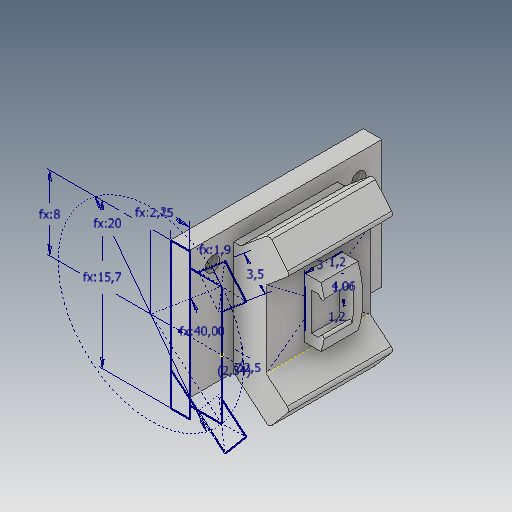
# Autodesk Inventor part: IMU_Fixation
Saved by Autodesk Inventor 2021.4 (Build 254397000, 397)
## iProperties
Created: 2022-04-26
Part Number: IMU_Fixation
Material: Generisch
Document SubType Name: Modeling
Designer: alexw
Density: 1 g/cm^3
Appearance: Vorgabe
Mass: 1.28857 g
Surface Area: 10.9165 cm^2
Volume: 1.28857 cm^3
SledWidth: 3,500 mm
SledDepth: 1,900 mm
Author: alexw
Autodesk Inventor part; units mm, degrees
ref_plane "YZ Plane" through (0, 0, 0) normal (1, 0, 0) x (0, 1, 0)
sketch "Sketch1" plane through (0, 0, 0) normal (0, 0, 1) x (1, 0, 0)
  line L0 (-1, 8) -> (1, 8)
  line L1 (1, 8) -> (1, -7.7)
  line L2 (1, -7.7) -> (-1, -7.7)
  line L3 (-1, -7.7) -> (-1, 8)
  line L4 (-1, 0) -> (1, 0) construction
  circle A0 centre (-3.15, 0) radius 10 construction
  line L5 (1, -6.4279) -> (4.5104, -6.4279)
  line L6 (4.5104, -6.4279) -> (4.5104, 6.4279)
  line L7 (4.5104, 6.4279) -> (1, 6.4279)
  line L8 (1, 6.4279) -> (1, -6.4279)
  line L9 (-3.15, 0) -> (4.5104, 6.4279) construction
  line L10 (-3.15, 0) -> (4.5104, -6.4279) construction
  line L11 (4.1798, 3.866) -> (7.0908, 6.3086) construction
  line L12 (7.0908, 6.3086) -> (4.8411, 8.9898)
  line L13 (4.8411, 8.9898) -> (1.9301, 6.5472) construction
  line L14 (1.9301, 6.5472) -> (4.1798, 3.866) construction
  line L15 (4.1798, 3.866) -> (4.8411, 8.9898) construction
  line L16 (7.0908, 6.3086) -> (1.9301, 6.5472) construction
  line L17 (4.1798, -3.866) -> (7.0908, -6.3086) construction
  line L18 (7.0908, -6.3086) -> (4.8411, -8.9898)
  line L19 (4.8411, -8.9898) -> (1.9301, -6.5472) construction
  line L20 (1.9301, -6.5472) -> (4.1798, -3.866) construction
  line L21 (4.1798, -3.866) -> (4.8411, -8.9898) construction
  line L22 (7.0908, -6.3086) -> (1.9301, -6.5472) construction
  line L23 (4.8411, 8.9898) -> (1.7879, 6.4279)
  line L24 (7.0908, 6.3086) -> (4.5104, 4.1434)
  line L25 (7.0908, -6.3086) -> (4.5104, -4.1434)
  line L26 (4.8411, -8.9898) -> (1.7879, -6.4279)
  line L27 (1, -6.4279) -> (1.7879, -6.4279)
  line L28 (1, -5.7667) -> (1, -6.4279)
  line L29 (1.7879, -6.4279) -> (-1, -4.0885)
  line L30 (6.85, 0) -> (-3.15, 0) construction
  point P0 (0, 0)
  point P1 (0, 0)
  point P2 (1.7879, 6.4279)
  point P3 (1, 6.4279)
  point P4 (1, -6.4279)
  point P5 (1.7879, -6.4279)
  point P6 (1, -5.7667)
  point P7 (6.7716, 1.25)
  dimension "d0" = 15.7
  dimension "d3" = 20
  dimension "SledAngle" = 40
  dimension "SledWidth" = 3.5
  dimension "SledDepth" = 1.9
  dimension "d7" = 2
  dimension "d30" = 2.15
  dimension "d74" = 8
  dimension "d88" = 2.3396
  dimension "d89" = 2.5
  constraints: 62 end point, 14 point on line, 7 parallel, 6 midpoint, 5 perpendicular, 4 horizontal, 4 symmetric about line, 3 point on circle, 1 centre point, 1 coincident
  measures "d0" distance of L2.end L0.start
  measures "d3" diameter of A0
  measures "SledAngle" angle of L4 L9
  measures "SledWidth" distance between parallel lines of L11 L13
  measures "SledDepth" distance from line of L12 L6.end
  measures "d7" distance of L0.start L0.end
  measures "d30" distance from line of L3 L9.start
  measures "d74" distance between parallel lines of L0 L4
  measures "d88" distance edge to line of A0 L6
  measures "d89" diameter of point (6.772, 1.25) L30
extrude "Extrusion1" add sketch "Sketch1" against normal blind 20.8 contours L0 L1 L29 L3
ref_plane "Work Plane1" through (0, 0, -4.8) normal (0, 0, 1) x (1, 0, 0)
ref_plane "Work Plane2" through (0, 0, -16) normal (0, 0, -1) x (-1, 0, 0)
extrude "Sled1" add sketch "Sketch1" against normal blind 3 from surface at -4.8 contours L7 L6 L5 L29 L1 | L23 L12 L24 L6 L7 | L5 L6 L25 L18 L26
extrude "Extrusion8" add sketch "Sketch1" along normal blind 3 from surface at -16 contours L7 L6 L5 L29 L1 | L23 L12 L24 L6 L7 | L5 L6 L25 L18 L26
sketch "Sketch4" plane through (-1, -4.0885, 0) normal (-1, 0, 0) x (0, 0, 1)
  line L0 (-24.96, 4.0885) -> (4.16, 4.0885) construction
  line L1 (-18.3, 9.5885) -> (-2.5, 9.5885) construction
  line L2 (0, 12.0885) -> (-20.8, 12.0885) construction
  line L3 (-10.4, 12.0885) -> (-10.4, 9.5885) construction
  point P0 (0, 4.0885)
  point P1 (-2.5, -1.4115)
  point P2 (-18.3, -1.4115)
  dimension "d18" = 5.5
  dimension "d19" = 15.8
  constraints: 4 end point, 2 midpoint, 2 symmetric about line, 1 horizontal, 1 vertical
  measures "d18" distance from line of L0 L1.end
  measures "d19" distance of L1.end L1.start
hole "Hole1" at (-1, 5.5, -18.3) at (-1, 5.5, -2.5) direction (1, 0, 0) diameter 1.567 depth 2 thread size "M2x0.4" class "6H" standard "ISO Metric profile"
fillet "Fillet2" radius 0.4 8 edges at (4.8411, 8.9898, -6.3) (7.0908, 6.3086, -6.3) (7.0908, -6.3086, -6.3) (4.8411, -8.9898, -6.3) (4.8411, -8.9898, -14.5) (7.0908, -6.3086, -14.5) (4.8411, 8.9898, -14.5) (7.0908, 6.3086, -14.5)
sketch "Sketch10" plane through (1.7879, 6.4279, -7.8) normal (0, 0, -1) x (-1, 0, 0)
  arc A0 (-3.3102, -15.1112) -> (-2.7467, -15.1605) centre (-3.0038, -14.8541) ccw projected
  line L0 (-2.7467, -15.1605) -> (0.7879, -12.1946) projected
  line L1 (0.7879, -12.1946) -> (0.7879, 0) projected
  line L2 (0.7879, 0) -> (0, 0) projected
  line L3 (0, 0) -> (-2.7467, 2.3048) projected
  arc A1 (-2.7467, 2.3048) -> (-3.3102, 2.2555) centre (-3.0038, 1.9983) ccw projected
  line L4 (-3.3102, 2.2555) -> (-5.0458, 0.1871) projected
  arc A2 (-5.0458, 0.1871) -> (-4.9965, -0.3764) centre (-4.7393, -0.07) ccw projected
  line L5 (-4.9965, -0.3764) -> (-2.7225, -2.2845) projected
  line L6 (-2.7225, -2.2845) -> (-2.7225, -10.5713) projected
  line L7 (-2.7225, -10.5713) -> (-4.9965, -12.4794) projected
  arc A3 (-4.9965, -12.4794) -> (-5.0458, -13.0429) centre (-4.7393, -12.7858) ccw projected
  line L8 (-5.0458, -13.0429) -> (-3.3102, -15.1112) projected
  point P0 (1.7879, -6.4279)
extrude "Extrusion14" add sketch "Sketch10" along normal up to surface (5.2 mm away)
sketch "Sketch11" plane through (4.5104, -4.1434, -4.8) normal (1, 0, 0) x (0, 0, -1)
  line L0 (11.2, 0) -> (0, 0) construction
  line L1 (11.2, 8.2868) -> (0, 8.2868) construction
  line L2 (0, 0) -> (11.2, 8.2868) construction
  line L3 (0, 8.2868) -> (11.2, 0) construction
  line L4 (4.1, 6.1734) -> (7.1, 6.1734)
  line L5 (7.1, 6.1734) -> (7.1, 2.1134)
  line L6 (7.1, 2.1134) -> (4.1, 2.1134)
  line L7 (4.1, 2.1134) -> (4.1, 6.1734)
  line L8 (4.1, 6.1734) -> (7.1, 2.1134) construction
  line L9 (7.1, 6.1734) -> (4.1, 2.1134) construction
  line L10 (7.1, 6.1734) -> (8.1, 6.1734)
  line L11 (8.1, 6.1734) -> (8.1, 2.1134)
  line L12 (8.1, 2.1134) -> (7.1, 2.1134)
  line L13 (7.1, 2.1134) -> (7.1, 6.1734)
  line L14 (7.1, 6.1734) -> (8.1, 6.1734)
  line L15 (8.1, 6.1734) -> (8.1, 7.3734)
  line L16 (8.1, 7.3734) -> (7.1, 7.3734)
  line L17 (7.1, 7.3734) -> (7.1, 6.1734)
  line L18 (7.1, 2.1134) -> (8.1, 2.1134)
  line L19 (8.1, 2.1134) -> (8.1, 0.9134)
  line L20 (8.1, 0.9134) -> (7.1, 0.9134)
  line L21 (7.1, 0.9134) -> (7.1, 2.1134)
  point P0 (-4.8, 4.1434)
  point P1 (5.6, 4.1434)
  point P2 (7.1, 2.1134)
  point P3 (8.1, 2.1134)
  point P4 (8.1, 6.1734)
  dimension "d90" = 4.06
  dimension "d91" = 3
  dimension "d100" = 1
  dimension "d103" = 1.2
  dimension "d104" = 1.2
  constraints: 40 end point, 8 parallel, 4 horizontal, 4 perpendicular, 3 collinear, 3 midpoint
  measures "d90" distance between parallel lines of L4 L6
  measures "d91" distance between parallel lines of L5 L7
  measures "d100" distance between parallel lines of L11 L5
  measures "d103" distance between parallel lines of L16 L10
  measures "d104" distance between parallel lines of L12 L20
extrude "Extrusion15" add sketch "Sketch11" along normal blind 0.69 contours L4 L5 L6 L7
sketch "Sketch12" plane through (4.5104, -2.03, -8.9) normal (0, 0, 1) x (1, 0, 0)
  line L0 (0, 4.06) -> (0.69, 4.06) construction
  line L1 (1.5, 4.06) -> (2.26, 3.2889)
  circle A0 centre (-7.6604, 2.03) radius 10 construction
  arc A1 (2.26, 3.2889) -> (1.8035, 5.26) centre (-7.6604, 2.03) ccw
  line L2 (1.8035, 5.26) -> (0, 5.26)
  line L3 (0, -2.1134) -> (0, 6.1734) construction
  line L4 (0, 5.26) -> (0, 4.06)
  line L5 (1.5, 4.06) -> (0, 4.06)
  line L6 (0.69, 0) -> (0.69, 4.06) construction
  line L7 (0.69, 2.03) -> (2.3396, 2.03) construction
  line L8 (0, 0) -> (0.69, 0) construction
  line L9 (1.5, 0) -> (2.26, 0.7711)
  arc A2 (1.8035, -1.2) -> (2.26, 0.7711) centre (-7.6604, 2.03) ccw
  line L10 (1.8035, -1.2) -> (0, -1.2)
  line L11 (0, -1.2) -> (0, 0)
  line L12 (1.5, 0) -> (0, 0)
  point P0 (-4.5104, 2.03)
  dimension "d94" = 1.57
  dimension "d95" = 1.2
  dimension "d96" = 0.81
  constraints: 20 end point, 7 point on circle, 5 symmetric about line, 2 centre point, 2 collinear, 1 concentric, 1 horizontal, 1 midpoint, 1 perpendicular, 1 point on line, 1 other
  measures "d94" distance from line of L1.end L6
  measures "d95" distance between parallel lines of L2 L5
  measures "d96" horizontal distance of L1.start L7.start
extrude "Extrusion16" add sketch "Sketch12" against normal up to surface (3 mm away)
fillet "Fillet3" radius 0.2 2 edges at (6.7704, 1.2589, -10.4) (6.7704, -1.2589, -10.4)
extrude "Extrusion17" add sketch "Sketch11" along normal up to surface contours L10 L11 L12 L5 | L17 L16 L15 L10 | L12 L19 L20 L21 round surface about axis through (-3.15, 0, -8.9) along (0, 0, -1) radius 10 far side no
thicken "Thicken1" operation add thickness 0.1 both sides no extend neighbours yes toward (1, 0, 0) faces at (5.2004, -0.6767, -10.9)
equation "\"d0\" = d74 + B_Frame_Y_bottom_1"
equation "\"d3\" = InnerDia_IMU"
equation "\"SledAngle\" = SlideAngle"
equation "\"d30\" = bno055_chip_Dist_height"
equation "\"d74\" = B_Frame_Y_top"
equation "\"Hole_Dist\" = 8"
equation "\"BoardLength\" = 20.8"
equation "\"Hole_Height\" = 5.5"
equation "\"Fix_Hole_Width\" = 15.8"
equation "\"Contact_Dist\" = 6.08677"
equation "\"B_Frame_Y_bottom_1\" = 7.7"
equation "\"InnerDia_IMU\" = 20"
equation "\"SlideAngle\" = 40deg"
equation "\"bno055_chip_Dist_height\" = 2.15"
equation "\"B_Frame_Y_top\" = 8"
body "Solid1"
